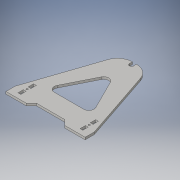
# Autodesk Inventor part: A8-0007
Saved by Autodesk Inventor 2016 SP2 (Build 200236200, 236)
## iProperties
Created: 2017-04-22
Part Number: A8-0007
Material: Generic
Document SubType Name: Modeling
Designer: EV
Density: 1 g/cm^3
Appearance: Default
Author: EV
Autodesk Inventor part; units mm, degrees
ref_plane "YZ Plane" through (0, 0, 0) normal (1, 0, 0) x (0, 1, 0)
ref_plane "XZ Plane" through (0, 0, 0) normal (0, 1, 0) x (-1, 0, 0)
ref_plane "XY Plane" through (0, 0, 0) normal (0, 0, 1) x (1, 0, 0)
sketch "Sketch1" plane through (0, 0, 0) normal (0, 1, 0) x (-1, 0, 0)
  line L0 (77.5, 0) -> (37.5, 0)
  line L1 (37.5, 0) -> (27.5, -10)
  line L2 (27.5, -10) -> (-27.5, -10)
  line L3 (-27.5, -10) -> (-37.5, 0)
  line L4 (-37.5, 0) -> (-77.5, 0)
  line L5 (-77.5, 0) -> (-77.5, -18)
  line L6 (-77.5, -18) -> (-31.6982, -154.0969)
  line L7 (31.6982, -154.0969) -> (77.5, -18)
  line L8 (77.5, -18) -> (77.5, 0)
  line L9 (0, -164) -> (0, -10) construction
  arc A0 (4, -174) -> (31.6982, -154.0969) centre (4, -144.7754) ccw
  arc A1 (-31.6982, -154.0969) -> (-4, -174) centre (-4, -144.7754) ccw
  line L10 (31.6982, -154.0969) -> (25, -174) construction
  line L11 (25, -174) -> (-25, -174) construction
  line L12 (-25, -174) -> (-42.9022, -120.8048) construction
  line L13 (4, -174) -> (4, -168)
  line L14 (4, -168) -> (-4, -168) construction
  line L15 (-4, -168) -> (-4, -174)
  arc A2 (4, -168) -> (-4, -168) centre (0, -168) ccw
  line L16 (28.8197, -46) -> (-28.8197, -46)
  line L17 (-37.7639, -60.4721) -> (-8.9443, -118.1115)
  line L18 (8.9443, -118.1115) -> (37.7639, -60.4721)
  arc A3 (37.7639, -60.4721) -> (28.8197, -46) centre (28.8197, -56) ccw
  arc A4 (-8.9443, -118.1115) -> (8.9443, -118.1115) centre (0, -113.6393) ccw
  arc A5 (-28.8197, -46) -> (-37.7639, -60.4721) centre (-28.8197, -56) ccw
  line L19 (63.5, -40) -> (58, -40)
  line L20 (58, -40) -> (58, -29.5)
  line L21 (58, -29.5) -> (63.5, -29.5)
  line L22 (63.5, -29.5) -> (63.5, -40)
  line L23 (63.5, -20) -> (58, -20)
  line L24 (58, -20) -> (58, -9.5)
  line L25 (58, -9.5) -> (63.5, -9.5)
  line L26 (63.5, -9.5) -> (63.5, -20)
  line L27 (-58, -29.5) -> (-63.5, -29.5)
  line L28 (-63.5, -29.5) -> (-63.5, -40)
  line L29 (-63.5, -40) -> (-58, -40)
  line L30 (-58, -40) -> (-58, -29.5)
  line L31 (-58, -9.5) -> (-63.5, -9.5)
  line L32 (-63.5, -9.5) -> (-63.5, -20)
  line L33 (-63.5, -20) -> (-58, -20)
  line L34 (-58, -20) -> (-58, -9.5)
  line L35 (60.75, -29.5) -> (60.75, -20) construction
  line L36 (-60.75, -29.5) -> (-60.75, -20) construction
  point P0 (0, 0)
  point P1 (45, -46)
  point P2 (-45, -46)
  point P3 (0, -136)
  point P4 (0, -46)
  point P5 (60.75, -24.75)
  point P6 (-60.75, -24.75)
  dimension "d1" = 155
  dimension "d2" = 10
  dimension "d3" = 45
  dimension "d4" = 55
  dimension "d5" = 18
  dimension "d6" = 174
  dimension "d7" = 50
  dimension "d8" = 8
  dimension "d9" = 6
  dimension "d13" = 90
  dimension "d14" = 46
  dimension "d15" = 136
  dimension "d16" = 10
  dimension "d17" = 5.5
  dimension "d18" = 10.5
  dimension "d19" = 9.5
  dimension "d20" = 29.5
  dimension "d21" = 14
  constraints: 74 end point, 13 point on circle, 12 point on line, 10 tangent, 9 midpoint, 8 equal length, 8 horizontal, 8 parallel, 7 collinear, 7 perpendicular, 6 centre point, 5 vertical, 2 equal radius, 2 vertical alignment, 1 coincident, 2 other
  measures "d1" distance between parallel lines of L8 L5
  measures "d2" distance between parallel lines of L2 L0
  measures "d3" angle of L0 L1
  measures "d4" distance of L1.end L2.end
  measures "d5" distance of L7.end L0.start
  measures "d6" distance from line of point (0, 0) L11
  measures "d7" distance of L10.end L11.end
  measures "d8" distance between parallel lines of L15 L13
  measures "d9" distance between parallel lines of L11 L14
  measures "d13" distance of point (45, -46) point (-45, -46)
  measures "d14" distance from line of point (0, 0) L16
  measures "d15" distance of point (0, 0) point (0, -136)
  measures "d16" radius of A3
  measures "d17" distance of L24.end L25.end
  measures "d18" distance of L25.end L23.start
  measures "d19" distance between parallel lines of L0 L25
  measures "d20" distance between parallel lines of L0 L21
  measures "d21" distance between parallel lines of L8 L26
extrude "Extrusion1" add sketch "Sketch1" along normal blind 4.5
hole "Hole1" at (-60.75, 0, -24.75) at (60.75, 0, -24.75) direction (0, 1, 0) diameter 3.5 end through all
body "Solid1"
